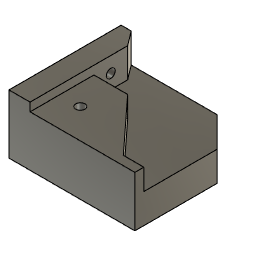
devansh1 v1 (Autodesk Fusion 360 design; units mm, degrees)
Autodesk Fusion 360 part; units mm, degrees
note: some values were not read from the file. Set by a fixed rule: which sketch regions a step uses.
sketch "Sketch1" plane through (0, 0, 0) normal (0, 0, 1) x (1, 0, 0)
  line L0 (0, 0) -> (174.2555, 0)
  line L1 (174.2555, 0) -> (174.2555, 132.964)
  line L2 (174.2555, 132.964) -> (0, 132.964)
  line L3 (0, 132.964) -> (0, 0)
  line L4 (138.7597, 132.964) -> (174.2555, 97.4682)
  line L5 (138.7597, 132.964) -> (188.9583, 132.964) construction
  dimension "d1" = 45
  constraint horizontal L0
  constraint vertical L1
  constraint horizontal L2
  constraint vertical L3
  constraint coincident L0.start L3.end
  constraint horizontal L5
  constraint coincident L2 L4.start
  constraint coincident L1 L4.end
  measures "d1" angle of L4 L5
extrude "Extrude1" add sketch "Sketch1" along normal blind 35 contours L0 L1 L2 L3 L4
extrude "Extrude2" cut 1 faces at (0, 88.6427, 11.6667) along direction (1, 0, 0) blind 25
sketch "Sketch2" plane through (0, 0, 35) normal (0, 0, 1) x (-1, 0, 0)
  line L0 (-25, -132.964) -> (-25, 0)
  line L1 (-25, 0) -> (-174.2555, 0)
  line L2 (-174.2555, 0) -> (-174.2555, -97.4682)
  line L3 (-174.2555, -97.4682) -> (-138.7597, -132.964)
  line L4 (-138.7597, -132.964) -> (-25, -132.964)
  line L5 (-25, -132.964) -> (-25, 0)
  line L6 (-50, 0) -> (-50, -110)
  line L7 (-50, -110) -> (-50, -115.7208)
  line L8 (-50, -115.7208) -> (-36.875, -132.964)
  constraint coincident L0.start L4.end
  constraint coincident L0.end L1.start
  constraint coincident L1 L6.start
  constraint perpendicular L1 L6
  constraint parallel L6 L7
  constraint coincident L4 L8.end
extrude "Extrude3" add sketch "Sketch2" along normal blind 35 contours L0 L1 L4 L5 L6 L7 L8
sketch "Sketch3" plane through (0, 0, 35) normal (0, 0, 1) x (-1, 0, 0)
  line L0 (-36.875, -132.964) -> (-50, -115.7208)
  line L1 (-50, -115.7208) -> (-50, 0)
  line L2 (-50, 0) -> (-174.2555, 0)
  line L3 (-174.2555, 0) -> (-174.2555, -97.4682)
  line L4 (-174.2555, -97.4682) -> (-138.7597, -132.964)
  line L5 (-138.7597, -132.964) -> (-36.875, -132.964)
  line L6 (-174.2555, -10.6135) -> (-155, -10.6135)
  line L7 (-50, 0) -> (-174.2555, 0)
  line L8 (-155, -10.6135) -> (-150, -10.6135)
  line L9 (-50, -75.7001) -> (-90, -75.7001)
  line L10 (-90, -75.7001) -> (-150, -10.6135)
  constraint coincident L3 L6.start
  constraint perpendicular L3 L6
  constraint coincident L1.end L2.start
  constraint coincident L2.end L3.start
  constraint parallel L6 L8
  constraint coincident L1 L9.start
  constraint perpendicular L1 L9
extrude "Extrude4" add sketch "Sketch3" along normal blind 25 contours L1 L2 L3 L6 L7 L8 L9 L10
sketch "Sketch4" plane through (50, 0, 0) normal (1, 0, 0) x (0, 1, 0)
  line L0 (75.7001, 60) -> (75.7001, 35)
  line L1 (75.7001, 35) -> (115.7208, 35)
  line L2 (115.7208, 35) -> (115.7208, 70)
  line L3 (115.7208, 70) -> (0, 70)
  line L4 (0, 70) -> (0, 60)
  line L5 (0, 60) -> (75.7001, 60)
  circle A0 centre (95.7105, 51.6698) radius 5.2582
extrude "Extrude5" cut sketch "Sketch4" against normal blind 50 contours A0
sketch "Sketch5" plane through (0, 0, 60) normal (0, 0, 1) x (-1, 0, 0)
  line L0 (-174.2555, -10.6135) -> (-150, -10.6135)
  line L1 (-150, -10.6135) -> (-90, -75.7001)
  line L2 (-90, -75.7001) -> (-50, -75.7001)
  line L3 (-50, -75.7001) -> (-50, 0)
  line L4 (-50, 0) -> (-174.2555, 0)
  line L5 (-174.2555, 0) -> (-174.2555, -10.6135)
  circle A0 centre (-74.3342, -35.2984) radius 5.4818
extrude "Extrude6" cut sketch "Sketch5" against normal blind 150 contours A0
